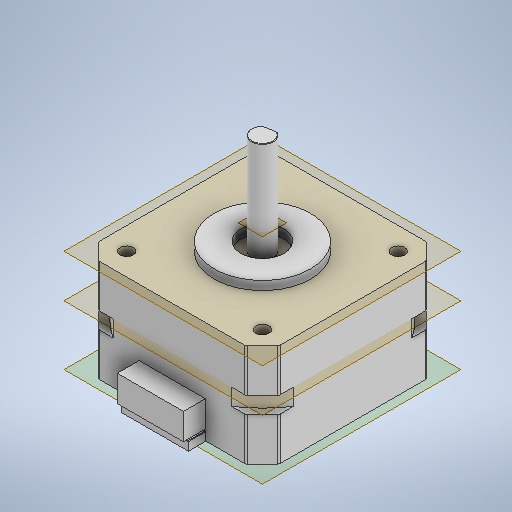
# Autodesk Inventor part: stepper_motor
Saved by Autodesk Inventor 2025.1 (Build 291241000, 241)
## iProperties
Created: 2024-11-21
Part Number: stepper_motor
Material: 一般
Document SubType Name: Modeling
Designer: dell
Density: 1 g/cm^3
Appearance: 既定
Author: dell
Autodesk Inventor part; units mm, degrees
ref_plane "YZ Plane" through (0, 0, 0) normal (1, 0, 0) x (0, 1, 0)
ref_plane "XZ Plane" through (0, 0, 0) normal (0, 1, 0) x (-1, 0, 0)
ref_plane "XY Plane" through (0, 0, 0) normal (0, 0, 1) x (1, 0, 0)
sketch "スケッチ1" plane through (0, 0, 0) normal (0, 1, 0) x (-1, 0, 0)
  line L0 (41.0243, -3.6426) -> (37.5574, -0.1757)
  line L1 (41.0243, -37.5574) -> (37.5574, -41.0243)
  line L2 (3.6426, -0.1757) -> (0.1757, -3.6426)
  line L3 (0.1757, -37.5574) -> (3.6426, -41.0243)
  line L4 (0, -37.1331) -> (0, -4.0669)
  line L5 (37.1331, -41.2) -> (4.0669, -41.2)
  line L6 (41.2, -4.0669) -> (41.2, -37.1331)
  line L7 (37.1331, 0) -> (4.0669, 0)
  arc A0 (41.2, -4.0669) -> (41.0243, -3.6426) centre (40.6, -4.0669) ccw
  arc A1 (37.5574, -0.1757) -> (37.1331, 0) centre (37.1331, -0.6) ccw
  arc A2 (4.0669, 0) -> (3.6426, -0.1757) centre (4.0669, -0.6) ccw
  arc A3 (0.1757, -3.6426) -> (0, -4.0669) centre (0.6, -4.0669) ccw
  arc A4 (0, -37.1331) -> (0.1757, -37.5574) centre (0.6, -37.1331) ccw
  arc A5 (3.6426, -41.0243) -> (4.0669, -41.2) centre (4.0669, -40.6) ccw
  arc A6 (37.1331, -41.2) -> (37.5574, -41.0243) centre (37.1331, -40.6) ccw
  arc A7 (41.0243, -37.5574) -> (41.2, -37.1331) centre (40.6, -37.1331) ccw
  line L8 (25.8, 0) -> (15.4, 0)
  point P0 (0, 0)
  point P1 (41.2, -3.8184)
  point P2 (37.3816, 0)
  point P3 (39.2908, -1.9092)
  point P4 (37.3816, -41.2)
  point P5 (41.2, -37.3816)
  dimension "d2" = 5.4
  dimension "d3" = 5.4
  dimension "d4" = 0.6
  constraints: 18 end point, 16 point on circle, 16 tangent, 8 centre point, 7 equal radius, 6 point on line, 2 perpendicular, 1 horizontal, 1 midpoint, 1 vertical
  measures "d2" distance of point (41.2, -3.818) point (37.382, 0)
  measures "d3" distance of point (41.2, -37.382) point (37.382, -41.2)
  measures "d4" radius of A0
extrude "押し出し1" add sketch "スケッチ1" along normal blind 9.8
sketch "スケッチ2" plane through (0, 9.8, 0) normal (0, 1, 0) x (1, 0, 0)
  line L0 (-41.2, 37.1331) -> (-41.2, 4.0669) projected
  line L1 (-41.0243, 3.6426) -> (-37.5574, 0.1757) projected
  line L2 (-4.0669, 41.2) -> (-37.1331, 41.2) projected
  line L3 (0, 4.0669) -> (0, 37.1331) projected
  line L4 (-37.1331, 0) -> (-4.0669, 0) projected
  line L5 (0, 34.1568) -> (0, 7.099)
  line L6 (-7.099, 0) -> (-34.1289, 0)
  line L7 (-41.2, 7.0711) -> (-41.2, 34.1568)
  line L8 (-37.5574, 41.0243) -> (-41.0243, 37.5574) projected
  line L9 (-3.6426, 0.1757) -> (-0.1757, 3.6426) projected
  arc A0 (-41.2, 7.0711) -> (-34.1289, 0) centre (-20.6, 20.6) ccw
  arc A1 (-7.071, 0) -> (0, 7.071) centre (-20.6, 20.6) ccw
  arc A2 (0, 34.1289) -> (-7.0711, 41.2) centre (-20.6, 20.6) ccw
  arc A3 (-34.1289, 41.2) -> (-41.2, 34.1289) centre (-20.6, 20.6) ccw
  line L10 (-34.1289, 0) -> (-7.071, 0)
  line L11 (-41.2, 7.0711) -> (-41.2, 34.1289)
  line L12 (-34.1289, 41.2) -> (-7.0711, 41.2)
  line L13 (0, 34.1289) -> (0, 7.071)
  point P0 (0, 0)
  point P1 (0, 40.8633)
  point P2 (-37.6645, 3.5355)
  point P3 (0, 34.1289)
  point P4 (-41.2, 41.2)
  point P5 (-7.071, 0)
  point P6 (0, 7.071)
  dimension "d8" = 10
  dimension "d9" = 10
  constraints: 14 end point, 11 point on line, 8 point on circle, 5 collinear, 4 centre point, 4 coincident, 1 perpendicular
  measures "d8" distance of L7.start L6.end
  measures "d9" distance of L11.end L12.start
extrude "押し出し2" add sketch "スケッチ2" along normal blind 3.8
ref_plane "作業平面1" through (0, 13.6, 0) normal (0, 1, 0) x (1, 0, 0)
sketch "スケッチ4" plane through (0, 13.6, 0) normal (0, 1, 0) x (1, 0, 0)
  line L0 (-4.0669, 0) -> (-37.1331, 0)
  line L1 (-41.2, 4.0669) -> (-41.2, 37.1331)
  line L2 (-37.1331, 41.2) -> (-4.0669, 41.2)
  line L3 (0, 37.1331) -> (0, 4.0669)
  line L4 (-41.0243, 3.6426) -> (-37.5574, 0.1757) projected
  line L5 (-41.0243, 3.6426) -> (-37.5574, 0.1757)
  line L6 (-0.1757, 37.5574) -> (-3.6426, 41.0243) projected
  line L7 (-3.6426, 41.0243) -> (-0.1757, 37.5574)
  line L8 (-3.6426, 0.1757) -> (-0.1757, 3.6426) projected
  line L9 (-0.1757, 3.6426) -> (-3.6426, 0.1757)
  line L10 (-37.5574, 41.0243) -> (-41.0243, 37.5574) projected
  line L11 (-37.5574, 41.0243) -> (-41.0243, 37.5574)
  arc A0 (-37.1331, 41.2) -> (-37.5574, 41.0243) centre (-37.1331, 40.6) ccw
  arc A1 (-41.0243, 37.5574) -> (-41.2, 37.1331) centre (-40.6, 37.1331) ccw
  line L12 (-41.0243, 3.6426) -> (-37.5574, 0.1757)
  arc A2 (-41.2, 4.0669) -> (-41.0243, 3.6426) centre (-40.6, 4.0669) ccw
  arc A3 (-37.5574, 0.1757) -> (-37.1331, 0) centre (-37.1331, 0.6) ccw
  arc A4 (-3.6426, 41.0243) -> (-4.0669, 41.2) centre (-4.0669, 40.6) ccw
  arc A5 (0, 37.1331) -> (-0.1757, 37.5574) centre (-0.6, 37.1331) ccw
  line L13 (-0.1757, 3.6426) -> (-3.6426, 0.1757)
  arc A6 (-0.1757, 3.6426) -> (0, 4.0669) centre (-0.6, 4.0669) ccw
  arc A7 (-4.0669, 0) -> (-3.6426, 0.1757) centre (-4.0669, 0.6) ccw
  point P0 (0, 0)
  point P1 (-41.2, 41.2)
  point P2 (-41.2, 0)
  point P3 (0, 41.2)
  point P4 (-41.0243, 37.5574)
  point P5 (-0.1757, 3.6426)
  dimension "d16" = 41.2
  dimension "d17" = 41.2
  dimension "d18" = 0.6
  dimension "d19" = 0.6
  dimension "d20" = 0.6
  dimension "d21" = 0.6
  dimension "d22" = 0.6
  constraints: 21 end point, 17 point on line, 16 point on circle, 16 tangent, 8 centre point, 7 equal length, 3 equal radius, 1 horizontal, 1 perpendicular
  measures "d16" distance of point (-41.2, 41.2) point (0, 41.2)
  measures "d17" distance of point (-41.2, 0) point (-41.2, 41.2)
  measures "d18" radius of A0
  measures "d19" radius of A2
  measures "d20" radius of A4
  measures "d21" radius of A6
  measures "d22" radius of A7
extrude "押し出し3" add sketch "スケッチ4" along normal blind 9.8
ref_plane "作業平面2" through (0, 0, 0) normal (0, -1, 0) x (1, 0, 0)
sketch "スケッチ5" plane through (0, 0, 0) normal (0, -1, 0) x (1, 0, 0)
  line L0 (-37.1331, 0) -> (-4.0669, 0) projected
  line L1 (-37.1331, 0) -> (-4.0669, 0) projected
  line L2 (-28.3, 0) -> (-12.9, 0)
  line L3 (-12.9, 0) -> (-12.9, 3.9)
  line L4 (-13, 4) -> (-28.2, 4)
  line L5 (-28.3, 3.9) -> (-28.3, 0)
  arc A0 (-28.2, 4) -> (-28.3, 3.9) centre (-28.2, 3.9) ccw
  arc A1 (-12.9, 3.9) -> (-13, 4) centre (-13, 3.9) ccw
  point P0 (0, 0)
  point P1 (-15.4, 0)
  point P2 (-12.9, 4)
  point P3 (-28.3, 4)
  point P4 (-28.3, 0)
  point P5 (-12.9, 0)
  point P6 (-20.6, 0)
  point P7 (-20.6, 0)
  dimension "d35" = 0.1
  dimension "d77" = 15.4
  constraints: 8 end point, 4 point on circle, 4 point on line, 4 tangent, 2 centre point, 2 parallel, 1 equal radius, 1 horizontal, 1 midpoint, 1 perpendicular
  measures "d35" radius of A0
  measures "d77" distance between parallel lines of L3 L5
extrude "押し出し4" add sketch "スケッチ5" against normal blind 2
fillet "フィレット1" radius 0.1 5 edges at (-12.9, 2, 1.95) (-20.6, 2, 4) (-28.2707, 2, 3.9707) (-28.3, 2, 1.95) (-12.9293, 2, 3.9707)
ref_plane "作業平面3" through (0, 23.4, 0) normal (0, 1, 0) x (1, 0, 0)
sketch "スケッチ6" plane through (0, 23.4, 0) normal (0, 1, 0) x (1, 0, 0)
  line L0 (-41.2, 37.1331) -> (-41.2, 4.0669) projected
  line L1 (-4.0669, 41.2) -> (-37.1331, 41.2) projected
  line L2 (0, 4.0669) -> (0, 37.1331) projected
  line L3 (-37.1331, 0) -> (-4.0669, 0) projected
  circle A0 centre (-36.1, 5.1) radius 1.5
  circle A1 centre (-36.1, 36.1) radius 1.5
  circle A2 centre (-5.1, 36.1) radius 1.5
  circle A3 centre (-5.1, 5.1) radius 1.5
  point P0 (0, 0)
  dimension "d39" = 5.1
  dimension "d40" = 5.1
  dimension "d41" = 5.1
  dimension "d42" = 5.1
  dimension "d43" = 5.1
  dimension "d44" = 5.1
  dimension "d45" = 5.1
  dimension "d46" = 5.1
  dimension "d47" = 3
  dimension "d48" = 3
  dimension "d49" = 3
  dimension "d50" = 3
  constraints: 4 centre point, 4 coincident
  measures "d39" distance from line of L0 point (-36.1, 36.1)
  measures "d40" distance from line of L1 point (-36.1, 36.1)
  measures "d41" distance from line of L2 point (-5.1, 36.1)
  measures "d42" distance from line of L1 point (-5.1, 36.1)
  measures "d43" distance from line of L2 point (-5.1, 5.1)
  measures "d44" distance from line of L3 point (-5.1, 5.1)
  measures "d45" distance from line of L3 point (-36.1, 5.1)
  measures "d46" distance from line of L0 point (-36.1, 5.1)
  measures "d47" diameter of A0
  measures "d48" diameter of A1
  measures "d49" diameter of A2
  measures "d50" diameter of A3
hole "穴1" at (-36.1, 23.4, -5.1) at (-36.1, 23.4, -36.1) at (-5.1, 23.4, -36.1) at (-5.1, 23.4, -5.1) direction (0, -1, 0) diameter 3 depth 4.5
sketch "スケッチ7" plane through (0, 23.4, 0) normal (0, 1, 0) x (1, 0, 0)
  circle A0 centre (-20.6, 20.6) radius 11
  circle A1 centre (-20.6, 20.6) radius 4.9
  point P0 (0, 0)
  dimension "d58" = 22
  dimension "d59" = 9.8
  constraints: 2 centre point, 2 coincident
  measures "d58" diameter of A0
  measures "d59" diameter of A1
extrude "押し出し5" add sketch "スケッチ7" along normal blind 2
sketch "スケッチ8" plane through (-20.6, 23.4, -20.6) normal (0, 1, 0) x (1, 0, 0)
  circle A0 centre (0, 0) radius 4.9 projected
  circle A1 centre (0, 0) radius 2.5
  point P0 (20.6, -20.6)
  dimension "d62" = 5
  constraints: 1 centre point, 1 coincident
  measures "d62" diameter of A1
extrude "押し出し6" add sketch "スケッチ8" along normal blind 5.6 contours A1
ref_plane "作業平面4" through (-20.6, 29, -20.6) normal (0, 1, 0) x (1, 0, 0)
sketch "スケッチ9" plane through (-20.6, 29, -20.6) normal (0, 1, 0) x (1, 0, 0)
  line L0 (-1.8244, 1.7093) -> (1.1301, 2.23)
  circle A0 centre (0, 0) radius 2.5 projected
  arc A1 (-1.8244, 1.7093) -> (1.1301, 2.23) centre (0, 0) ccw
  point P0 (20.6, -20.6)
  dimension "d67" = 3
  constraints: 4 point on circle, 2 end point, 1 centre point, 1 coincident
  measures "d67" distance of L0.start L0.end
extrude "押し出し7" add sketch "スケッチ9" along normal blind 17.4 contours L0 A0 picked at (-1.0191, 0.489)
fillet "フィレット2" radius 0.1 1 edges at (-20.1661, 46.4, -18.1379)
ref_plane "作業平面5" through (0, 2.3, 0) normal (0, 1, 0) x (1, 0, 0)
sketch "スケッチ10" plane through (0, 2.3, 0) normal (0, 1, 0) x (1, 0, 0)
  line L0 (-37.1331, 0) -> (-4.0669, 0) projected
  line L1 (-28.15, 0) -> (-13.05, 0)
  line L2 (-13.05, 0) -> (-13.05, -5)
  line L3 (-13.05, -5) -> (-28.15, -5)
  line L4 (-28.15, -5) -> (-28.15, 0)
  point P0 (0, 0)
  point P1 (-13.05, 0)
  point P2 (-13.05, 0)
  dimension "d74" = 5
  dimension "d80" = 15.1
  constraints: 8 end point, 2 parallel, 2 point on line, 1 horizontal, 1 perpendicular
  measures "d74" distance of L1.end L2.end
  measures "d80" distance of L2.end L3.end
extrude "押し出し8" add sketch "スケッチ10" along normal blind 6
sketch "スケッチ11" plane through (0, 0, 0) normal (0, -1, 0) x (1, 0, 0)
  circle A0 centre (-20.6, -20.6) radius 5
  point P0 (0, 0)
  dimension "d81" = 10
  constraints: 2 coincident, 1 centre point
  measures "d81" diameter of A0
hole "穴2" at (-20.6, 0, -20.6) direction (0, 1, 0) diameter 10 depth 3
